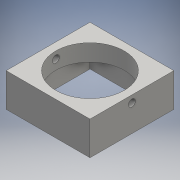
# Autodesk Inventor part: zwo camera support
Saved by Autodesk Inventor 2016 (Build 200138000, 138)
## iProperties
Created: 2015-12-13
Part Number: zwo camera support
Material: Generic
Document SubType Name: Modeling
Designer: roduino
Density: 1 g/cm^3
Appearance: Default
Author: roduino
Autodesk Inventor part; units mm, degrees
ref_plane "YZ Plane" through (0, 0, 0) normal (1, 0, 0) x (0, 1, 0)
ref_plane "XZ Plane" through (0, 0, 0) normal (0, 1, 0) x (-1, 0, 0)
ref_plane "XY Plane" through (0, 0, 0) normal (0, 0, 1) x (1, 0, 0)
sketch "Sketch1" plane through (0, 0, 0) normal (0, 0, 1) x (1, 0, 0)
  line L0 (-25, 25) -> (25, 25)
  line L1 (25, 25) -> (25, -25)
  line L2 (25, -25) -> (-25, -25)
  line L3 (-25, -25) -> (-25, 25)
  line L4 (30, 30) -> (-30, 30)
  line L5 (-30, 30) -> (-30, -30)
  line L6 (-30, -30) -> (30, -30)
  line L7 (30, -30) -> (30, 30)
  point P0 (0, 0)
  dimension "d0" = 50
  dimension "d1" = 50
  dimension "d2" = 25
  dimension "d3" = 25
  dimension "d4" = 5
  constraints: 16 end point, 4 parallel, 2 perpendicular, 1 horizontal, 3 other
  measures "d0" distance of L1.end L2.end
  measures "d1" distance of L0.end L1.end
  measures "d2" distance from line of point (0, 0) L0
  measures "d3" distance from line of point (0, 0) L3
  measures "d4" distance between parallel lines of L0 L4
extrude "Extrusion1" add sketch "Sketch1" along normal blind 12
sketch "Sketch2" plane through (0, 0, 12) normal (0, 0, 1) x (1, 0, 0)
  circle A0 centre (0, 0) radius 24.5
  line L0 (-30, 30) -> (-30, -30) projected
  line L1 (30, 30) -> (-30, 30) projected
  line L2 (30, -30) -> (30, 30) projected
  line L3 (-30, -30) -> (30, -30) projected
  dimension "d7" = 49
  constraints: 1 centre point, 1 coincident
  measures "d7" diameter of A0
extrude "Extrusion2" add sketch "Sketch2" along normal blind 12
hole "Hole1" at (21, 21, 12) direction (0, 0, 1) diameter 8 depth 5 tip angle 118
pattern_circular "Circular Pattern1" count 4 over 360 about axis through (0, 0, 12) along (0, 0, 1) of "Hole1"
sketch "Sketch3" plane through (-30, -30, 0) normal (-1, 0, 0) x (0, 0, 1)
  circle A0 centre (19, 30) radius 2.5
  line L0 (0, 60) -> (0, 0) projected
  line L1 (0, 0) -> (24, 0) projected
  point P0 (0, 30)
  dimension "d22" = 5
  dimension "d23" = 19
  dimension "d24" = 30
  constraints: 1 centre point
  measures "d22" diameter of A0
  measures "d23" distance from line of L0 A0.centre
  measures "d24" distance from line of L1 A0.centre
extrude "Extrusion3" cut sketch "Sketch3" against normal through all
equation "\"d2\" = 0.5 * d1"
equation "\"d3\" = 0.5 * d0"
body "Solid1"
